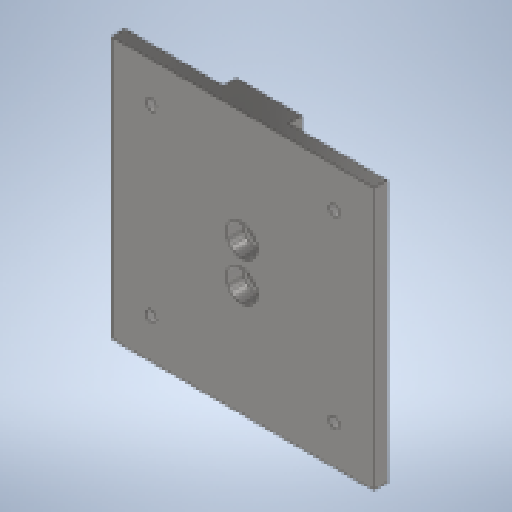
# Autodesk Inventor part: HCMUTE-CDT23-BAN_CAN_LOADCELL
Saved by Autodesk Inventor 2023 (Build 270158000, 158)
## iProperties
Created: 2023-10-14
Part Number: HCMUTE-CDT23-BAN_CAN_LOADCELL
Material: Stainless Steel
Document SubType Name: Modeling
Designer: havie
Density: 8 g/cm^3
Appearance: Steel - Polished
Mass: 916.805 g
Surface Area: 266.83 cm^2
Volume: 114.601 cm^3
Author: havie
Autodesk Inventor part; units mm, degrees
ref_plane "YZ Plane" through (0, 0, 0) normal (1, 0, 0) x (0, 1, 0)
ref_plane "XZ Plane" through (0, 0, 0) normal (0, 1, 0) x (-1, 0, 0)
ref_plane "XY Plane" through (0, 0, 0) normal (0, 0, 1) x (1, 0, 0)
sketch "Sketch4" plane through (0, 0, 0) normal (0, 0, 1) x (1, 0, 0)
  line L0 (-50, 50) -> (50, 50)
  line L1 (50, 50) -> (50, -50)
  line L2 (50, -50) -> (-50, -50)
  line L3 (-50, -50) -> (-50, 50)
  line L4 (-50, 50) -> (50, -50) construction
  line L5 (50, 50) -> (-50, -50) construction
  point P0 (0, 0)
  dimension "d34" = 100
  dimension "d35" = 100
  constraints: 12 end point, 2 midpoint, 2 parallel, 1 horizontal, 1 perpendicular
  measures "d34" distance of L1.end L2.end
  measures "d35" distance of L0.end L1.end
extrude "Extrusion2" add sketch "Sketch4" along normal mid plane 5
sketch "Sketch5" plane through (-50, -50, 2.5) normal (0, -1, 0) x (1, 0, 0)
  line L0 (0, -5) -> (100, -5) projected
  line L1 (37.5, -5) -> (62.5, -5)
  line L2 (62.5, -5) -> (62.5, -10)
  line L3 (62.5, -10) -> (37.5, -10)
  line L4 (37.5, -10) -> (37.5, -5)
  line L5 (100, -5) -> (0, -5) projected
  point P0 (50, -2.5)
  point P1 (50, -5)
  point P2 (62.5, -7.5)
  point P3 (37.5, -7.5)
  point P4 (50, -5)
  dimension "d38" = 25
  dimension "d39" = 12.5
  dimension "d40" = 5
  constraints: 8 end point, 4 midpoint, 2 parallel, 1 horizontal, 1 perpendicular, 1 point on line, 1 vertical alignment
  measures "d38" distance of point (62.5, -7.5) point (37.5, -7.5)
  measures "d39" distance from line of point (50, -5) L4
  measures "d40" distance of L3.end L1.start
extrude "Extrusion3" add sketch "Sketch5" against normal up to surface (100 mm away)
sketch "Sketch6" plane through (0, 0, 2.5) normal (0, 0, 1) x (1, 0, 0)
  circle A0 centre (-0.5, 7.5) radius 2.4585 projected
  line L0 (-12.5, 13.5) -> (12.5, 13.5) projected
  circle A1 centre (-0.5, -7.5) radius 2.4585 projected
  point P0 (0, 0)
  constraints: 2 coincident
hole "Hole3" at (-0.5, -7.5, 2.5) at (-0.5, 7.5, 2.5) direction (0, 0, -1) diameter 7 depth 17.1 tip angle 118 counterbore diameter 12 counterbore depth 6
sketch "Sketch7" plane through (0, 0, 2.5) normal (0, 0, 1) x (1, 0, 0)
  line L0 (50, -50) -> (50, 50) projected
  line L1 (-50, -50) -> (50, -50) projected
  line L2 (50, 50) -> (-50, 50) projected
  line L3 (-50, 50) -> (-50, -50) projected
  point P0 (0, 0)
  point P1 (35, -35)
  point P2 (-35, -35)
  point P3 (-35, 35)
  point P4 (35, 35)
  dimension "d50" = 15
  dimension "d51" = 15
  dimension "d52" = 15
  dimension "d53" = 15
  constraints: 2 horizontal alignment, 2 vertical alignment
  measures "d50" distance from line of L0 point (35, -35)
  measures "d51" distance from line of L1 point (35, -35)
  measures "d52" distance from line of L2 point (35, 35)
  measures "d53" distance from line of L3 point (-35, -35)
hole "Hole4" at (35, -35, 2.5) at (-35, -35, 2.5) at (-35, 35, 2.5) at (35, 35, 2.5) direction (0, 0, -1) diameter 4.134 depth 14.2 tip angle 118 thread size "M5x0.8" class "6H" standard "ISO Metric profile"
sketch "Sketch1" plane through (0, 0, 0) normal (0, 1, 0) x (-1, 0, 0)
  line L0 (65, -7.5) -> (-65, -7.5)
  line L1 (-65, -7.5) -> (-65, -7.5)
  line L2 (-65, -7.5) -> (-65, -7.5)
  line L3 (-65, -7.5) -> (-65, 2.5)
  line L4 (-65, 2.5) -> (-35, 2.5)
  line L5 (-35, 2.5) -> (-35, -2.5)
  line L6 (-35, -2.5) -> (65, -2.5)
  line L7 (65, -2.5) -> (65, -7.5)
  point P0 (0, 0)
  dimension "d0" = 130
  dimension "d1" = 130
  dimension "d2" = 30
  dimension "d5" = 5
  dimension "d6" = 5
  dimension "d7" = 10
  dimension "d8" = 65
  dimension "d9" = 7.5
  constraints: 16 end point, 7 perpendicular, 1 horizontal
  measures "d0" distance between parallel lines of L3 L7
  measures "d1" distance of L0.start L0.end
  measures "d2" distance of L3.end L4.end
  measures "d5" distance between parallel lines of L6 L2
  measures "d6" distance between parallel lines of L6 L0
  measures "d7" distance between parallel lines of L2 L4
  measures "d8" distance from line of point (0, 0) L7
  measures "d9" distance from line of point (0, 0) L0
sketch "Sketch3" plane through (65, 40, -7.5) normal (0, 0, -1) x (-1, 0, 0)
  line L0 (0, 0) -> (130, 0) projected
  line L1 (0, -80) -> (0, 0) projected
  point P0 (65, -40)
  point P1 (65, -40)
  point P2 (12, -32.5)
  point P3 (12, -47.5)
  dimension "d23" = 15
  dimension "d25" = 32.5
  dimension "d26" = 12
  constraints: 1 vertical alignment
  measures "d23" distance of point (12, -32.5) point (12, -47.5)
  measures "d25" distance from line of L0 point (12, -32.5)
  measures "d26" distance from line of L1 point (12, -32.5)
body "Solid1"
body "Solid2"
